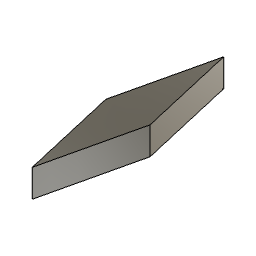
Rhombus (Autodesk Fusion 360 design; units mm, degrees)
Autodesk Fusion 360 part; units mm, degrees
sketch "Rhombus" plane through (0, 0, 0) normal (0, 0, 1) x (1, 0, 0)
  line L0 (2.54, 0) -> (5.08, -10.9977)
  line L1 (2.54, -21.9964) -> (0, -10.9982)
  line L2 (5.08, -10.9977) -> (2.54, -21.9964)
  line L3 (0, -10.9982) -> (2.54, 0)
extrude "Extrude1" add sketch "Rhombus" along normal blind 3.175
